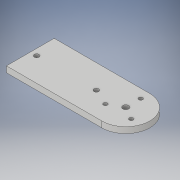
# Autodesk Inventor part: Robotics_PenMount
Saved by Autodesk Inventor 2019 (Build 230136000, 136)
## iProperties
Created: 2021-11-15
Part Number: Robotics_PenMount
Material: Generic
Document SubType Name: Modeling
Designer: colli
Density: 1 g/cm^3
Appearance: Default
Author: colli
Autodesk Inventor part; units mm, degrees
ref_plane "YZ Plane" through (0, 0, 0) normal (1, 0, 0) x (0, 1, 0)
ref_plane "XZ Plane" through (0, 0, 0) normal (0, 1, 0) x (-1, 0, 0)
ref_plane "XY Plane" through (0, 0, 0) normal (0, 0, 1) x (1, 0, 0)
sketch "Sketch1" plane through (0, 0, 0) normal (0, 1, 0) x (-1, 0, 0)
  circle A0 centre (0, 0) radius 19.05
  dimension "d0" = 38.1
  constraints: 1 centre point, 1 coincident
  measures "d0" diameter of A0
extrude "Extrusion1" add sketch "Sketch1" along normal blind 4.7625
sketch "Sketch2" plane through (0, 4.7625, 0) normal (0, 1, 0) x (1, 0, 0)
  circle A0 centre (0, 0) radius 2.3813
  circle A1 centre (0, 0) radius 19.05 projected
  circle A2 centre (-10.3056, -5.95) radius 1.5875
  circle A3 centre (0, 11.8999) radius 1.5875
  circle A4 centre (10.3056, -5.95) radius 1.5875
  dimension "d3" = 4.7625
  dimension "d4" = 3.175
  dimension "d5" = 3.175
  dimension "d6" = 3.175
  constraints: 4 centre point, 2 coincident
  measures "d3" diameter of A0
  measures "d4" diameter of A2
  measures "d5" diameter of A3
  measures "d6" diameter of A4
extrude "Extrusion2" cut sketch "Sketch2" against normal blind 4.7625 contours A0 | A2 | A3 | A4
sketch "Sketch3" plane through (0, 0, 0) normal (0, -1, 0) x (1, 0, 0)
  circle A0 centre (0, 0) radius 19.05 projected
  line L0 (0, -19.05) -> (0, 19.05)
  line L1 (0, 19.05) -> (-127, 19.05)
  line L2 (-127, 19.05) -> (-127, -19.05)
  line L3 (-127, -19.05) -> (0, -19.05)
  dimension "d9" = 127
  constraints: 8 end point, 2 parallel, 2 point on circle, 1 perpendicular, 1 vertical
  measures "d9" distance of L1.end L0.end
extrude "Extrusion3" add sketch "Sketch3" against normal blind 4.7625 contours A0 L3 L2 L1
sketch "Sketch4" plane through (0, 4.7625, 0) normal (0, 1, 0) x (1, 0, 0)
  line L0 (-127, 19.05) -> (-127, -19.05) projected
  line L1 (-127, 19.05) -> (-76.2, 19.05)
  line L2 (-76.2, 19.05) -> (-76.2, -19.05)
  line L3 (-76.2, -19.05) -> (-127, -19.05)
  line L4 (-127, -19.05) -> (-127, 19.05)
  point P0 (0, 0)
  dimension "d12" = 50.8
  constraints: 8 end point, 2 parallel, 1 horizontal, 1 perpendicular
  measures "d12" distance of L2.end L3.end
extrude "Extrusion4" cut sketch "Sketch4" against normal blind 25.4
sketch "Sketch5" plane through (0, 4.7625, 0) normal (0, 1, 0) x (1, 0, 0)
  line L0 (-76.2, 19.05) -> (-76.2, -19.05) projected
  line L1 (-76.2, 0) -> (-71.12, 0)
  circle A0 centre (-71.12, 0) radius 1.905
  line L2 (-71.12, 0) -> (-23.495, 0)
  circle A1 centre (-23.495, 0) radius 1.905
  point P0 (0, 0)
  dimension "d15" = 5.08
  dimension "d16" = 3.81
  dimension "d17" = 47.625
  dimension "d18" = 3.81
  constraints: 4 end point, 2 centre point, 2 coincident, 2 horizontal, 1 midpoint
  measures "d15" distance of L1.start L1.end
  measures "d16" diameter of A0
  measures "d17" distance of L2.start L2.end
  measures "d18" diameter of A1
extrude "Extrusion5" cut sketch "Sketch5" against normal blind 25.4
body "Solid1"
